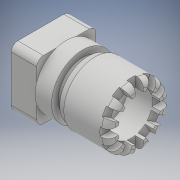
# Autodesk Inventor part: HbWristMountForChild
Saved by Autodesk Inventor 2018 (Build 220112000, 112)
## iProperties
Created: 2017-10-28
Part Number: HbWristMountForChild
Material: 一般
Document SubType Name: Modeling
Designer: sktom
Density: 1 g/cm^3
Appearance: 既定
Author: sktom
Autodesk Inventor part; units mm, degrees
ref_plane "YZ Plane" through (0, 0, 0) normal (1, 0, 0) x (0, 1, 0)
ref_plane "XZ Plane" through (0, 0, 0) normal (0, 1, 0) x (-1, 0, 0)
ref_plane "XY Plane" through (0, 0, 0) normal (0, 0, 1) x (1, 0, 0)
sketch "スケッチ1" plane through (0, 0, 0) normal (0, 0, 1) x (1, 0, 0)
  line L0 (0, 0) -> (0, 9.5)
  line L1 (0, 9.5) -> (5, 9.5)
  line L2 (5, 9.5) -> (5, 7.5)
  line L3 (5, 7.5) -> (6.75, 7.5)
  line L4 (6.75, 7.5) -> (6.75, 8.75)
  line L5 (6.75, 8.75) -> (8.75, 8.75)
  line L6 (8.75, 8.75) -> (8.75, 9.5)
  line L7 (8.75, 9.5) -> (22.25, 9.5)
  line L8 (22.25, 9.5) -> (22.25, 0)
  line L9 (22.25, 0) -> (0, 0)
  dimension "d0" = 5
  dimension "d1" = 9.5
  dimension "d2" = 1.75
  dimension "d3" = 2
  dimension "d4" = 13.5
  dimension "d5" = 7.5
  dimension "d6" = 8.75
  constraints: 20 end point, 8 perpendicular, 2 point on line, 1 vertical
  measures "d0" distance of L0.end L1.end
  measures "d1" distance of L0.start L0.end
  measures "d2" distance of L2.end L3.end
  measures "d3" distance of L4.end L5.end
  measures "d4" distance of L6.end L7.end
  measures "d5" distance between parallel lines of L9 L3
  measures "d6" distance between parallel lines of L9 L5
revolve "回転1" add sketch "スケッチ1" angle 360 about axis through (22.25, 0, 0) along (-1, 0, 0)
fillet "フィレット1" radius 2 1 edges at (22.25, -9.5, 0)
sketch "スケッチ2" plane through (22.25, 0, 0) normal (1, 0, 0) x (0, 0, -1)
  line L0 (-1.25, -9.5) -> (1.25, -9.5)
  line L1 (1.25, -9.5) -> (1.25, 9.5)
  line L2 (1.25, 9.5) -> (-1.25, 9.5)
  line L3 (-1.25, 9.5) -> (-1.25, -9.5)
  line L4 (-1.25, -9.5) -> (1.25, 9.5) construction
  line L5 (1.25, -9.5) -> (-1.25, 9.5) construction
  circle A0 centre (0, 0) radius 9.5 construction
  dimension "d9" = 2.5
  constraints: 12 end point, 2 midpoint, 2 parallel, 1 horizontal, 1 perpendicular, 1 tangent
  measures "d9" distance of L1.end L2.end
extrude "押し出し1" cut sketch "スケッチ2" against normal blind 2.5
pattern_circular "円形状パターン1" count 12 over 360 about axis through (15.5, 0, 0) along (1, 0, 0) of "押し出し1"
sketch "スケッチ3" plane through (22.25, 4.7801, 5.7793) normal (1, 0, 0) x (0, -0.5, -0.8660254)
  circle A0 centre (7.3951, -1.25) radius 6.5
  dimension "d15" = 13
  constraints: 1 centre point, 1 coincident
  measures "d15" diameter of A0
extrude "押し出し2" cut sketch "スケッチ3" against normal blind 10
sketch "スケッチ4" plane through (0, 0, 0) normal (-1, 0, 0) x (0, 0, 1)
  line L0 (-9, 9) -> (9, 9)
  line L1 (9, 9) -> (9, -9)
  line L2 (9, -9) -> (-9, -9)
  line L3 (-9, -9) -> (-9, 9)
  line L4 (-9, 9) -> (9, -9) construction
  line L5 (9, 9) -> (-9, -9) construction
  point P0 (0, 0)
  dimension "d19" = 18
  constraints: 12 end point, 2 midpoint, 2 parallel, 2 perpendicular, 1 horizontal
  measures "d19" distance of L0.end L1.end
extrude "押し出し3" add sketch "スケッチ4" along normal blind 7.8
fillet "フィレット2" radius 2 4 edges at (-3.9, 9, 9) (-3.9, 9, -9) (-3.9, -9, -9) (-3.9, -9, 9)
sketch "スケッチ5" plane through (-7.8, 0, 0) normal (-1, 0, 0) x (0, 0, 1)
  circle A0 centre (0, 0) radius 8.75 construction
  circle A1 centre (0, 0) radius 7 construction
  circle A2 centre (7, 0) radius 0.85
  circle A3 centre (-7, 0) radius 0.85
  point P0 (0, 0)
  dimension "d23" = 1.7
  dimension "d24" = 14
  constraints: 3 centre point, 2 horizontal alignment, 2 point on circle, 1 coincident, 1 equal radius
  measures "d23" diameter of A3
  measures "d24" diameter of A1
extrude "押し出し4" cut sketch "スケッチ5" against normal blind 12
